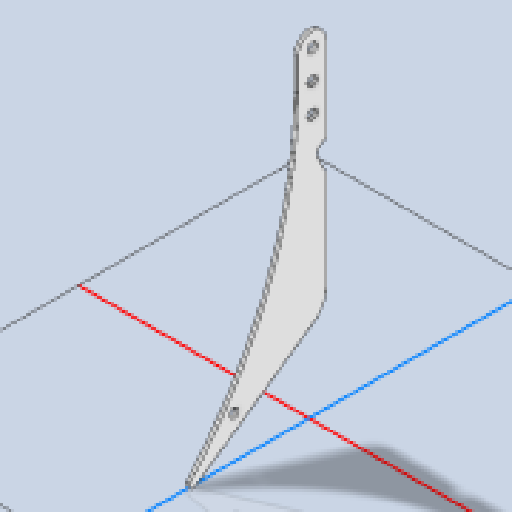
# Autodesk Inventor part: Ramp
Saved by Autodesk Inventor 2026 (Build 300175000, 175)
## iProperties
Created: 2025-04-08
Part Number: Ramp
Material: Acetal Resin, White
Document SubType Name: Modeling
Designer: avere
Density: 1.425 g/cm^3
Appearance: Smooth - White
Author: avere
Autodesk Inventor part; units mm, degrees
ref_plane "YZ Plane" through (0, 0, 0) normal (1, 0, 0) x (0, 1, 0)
ref_plane "XZ Plane" through (0, 0, 0) normal (0, 1, 0) x (-1, 0, 0)
ref_plane "XY Plane" through (0, 0, 0) normal (0, 0, 1) x (1, 0, 0)
sketch "main" plane through (0, 0, 0) normal (0, 0, 1) x (1, 0, 0)
  circle A0 centre (44.5304, -90.8931) radius 2.1844
  circle A1 centre (57.2304, -90.8931) radius 2.1844
  arc A2 (57.4426, -97.2395) -> (57.0183, -84.5466) centre (57.2304, -90.8931) ccw
  line L0 (57.0183, -84.5466) -> (42.9235, -84.5466)
  arc A3 (-82.6347, -36.8279) -> (42.9235, -84.5466) centre (42.9235, 104.498) ccw
  line L1 (57.4426, -97.2395) -> (-37.5462, -97.2395)
  line L2 (-47.9494, -91.8239) -> (-84.9895, -38.9252)
  arc A4 (-82.6347, -36.8279) -> (-84.9895, -38.9252) centre (-83.6891, -38.0147) ccw
  arc A5 (-47.9494, -91.8239) -> (-37.5462, -97.2395) centre (-37.5462, -84.5395) ccw
  circle A6 centre (31.8304, -90.8931) radius 2.1844
  point P0 (7.1274, -71.1865)
  point P1 (-94.5624, -25.2536)
  point P2 (-44.1574, -97.2395)
  dimension "d1" = 12.7
  dimension "d2" = 101.6
  dimension "d3" = 1.5875
  dimension "d4" = 12.7
  dimension "d7" = 64.5774
  dimension "d10" = 12.7
  dimension "d15" = 125
  dimension "d16" = 12.7
  measures "d1" diameter of A2
  measures "d2" distance of L1.start point (-44.157, -97.24)
  measures "d3" radius of A4
  measures "d4" radius of A5
  measures "d7" distance of L2.start L2.end
  measures "d10" distance of A0.centre A6.centre
  measures "d15" angle of L1 L2
  measures "d16" distance of A0.centre A1.centre
sketch "Sketch1" plane through (0, 0, 0) normal (1, 0, 0) x (0, 1, 0)
  arc A0 (-39.5025, -3.0335) -> (-42.7248, -2.0551) centre (-41.6029, -4.1554) ccw projected
  line L0 (-42.7248, -2.0551) -> (-52.3306, -7.186) projected
  line L1 (-39.5025, -3.0335) -> (-35.7298, -10.0964) projected
  circle A1 centre (-122.5435, 34.4996) radius 2.0955
  circle A2 centre (-12.7, 0) radius 2.1844
  circle A3 centre (0, 0) radius 2.1844
  arc A4 (0.2122, -6.3465) -> (-0.2122, 6.3465) centre (0, 0) ccw
  line L2 (-0.2122, 6.3465) -> (-14.307, 6.3465)
  arc A5 (-139.8652, 54.0652) -> (-14.307, 6.3465) centre (-14.307, 195.391) ccw
  line L3 (0.2122, -6.3465) -> (-94.7766, -6.3465)
  line L4 (-105.1799, -0.9309) -> (-142.2199, 51.9678)
  arc A6 (-139.8652, 54.0652) -> (-142.2199, 51.9678) centre (-140.9195, 52.8784) ccw
  arc A7 (-105.1799, -0.9309) -> (-94.7766, -6.3465) centre (-94.7766, 6.3535) ccw
  circle A8 centre (-25.4, 0) radius 2.1844
  point P0 (-50.7588, -6.3465)
  point P1 (-37.7329, -6.3465)
  constraints: 1 centre point, 3 other
extrude "Extrusion1" add sketch "Sketch1" along normal blind 1.5875 contours A0 L0 L3 A7 L4 A6 A5 L2 A4 L1
body "Solid1"
